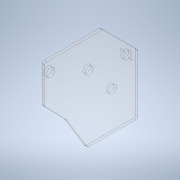
# Autodesk Inventor part: Intake-v2
Saved by Autodesk Inventor 2022 (Build 260153000, 153)
## iProperties
Created: 2022-01-09
Part Number: Intake-v2
Material: Generic
Document SubType Name: Modeling
Designer: merky
Density: 1 g/cm^3
Appearance: Polycarbonate - Clear
Mass: 272.104 g
Surface Area: 946.386 cm^2
Volume: 272.104 cm^3
Author: merky
Autodesk Inventor part; units mm, degrees
ref_plane "YZ Plane" through (0, 0, 0) normal (1, 0, 0) x (0, 1, 0)
ref_plane "XZ Plane" through (0, 0, 0) normal (0, 1, 0) x (-1, 0, 0)
ref_plane "XY Plane" through (0, 0, 0) normal (0, 0, 1) x (1, 0, 0)
sketch "Sketch1" plane through (0, 0, 0) normal (1, 0, 0) x (0, 1, 0)
  line L0 (348.73, -1.5913) -> (348.73, -164.0611)
  line L1 (346.8701, -168.5512) -> (220.7492, -294.6721)
  line L2 (216.2591, -296.532) -> (6.3382, -296.532)
  circle A0 centre (307.9632, 25.3963) radius 15.5575
  line L3 (348.73, -1.5913) -> (348.73, 40.2549)
  line L4 (-0.0118, -114.6125) -> (-0.0118, -290.182)
  arc A1 (5.4588, -108.3237) -> (-0.0118, -114.6125) centre (6.3382, -114.6125) ccw
  arc A2 (-0.0118, -290.182) -> (6.3382, -296.532) centre (6.3382, -290.182) ccw
  arc A3 (216.2591, -296.532) -> (220.7492, -294.6721) centre (216.2591, -290.182) ccw
  arc A4 (346.8701, -168.5512) -> (348.73, -164.0611) centre (342.38, -164.0611) ccw
  circle A5 centre (243.0455, -117.7246) radius 14.2875
  circle A6 centre (243.0455, -117.7246) radius 38.1 construction
  circle A7 centre (140.3051, -203.2037) radius 38.1 construction
  circle A8 centre (140.3051, -203.2037) radius 14.2875
  circle A9 centre (200.1626, -272.0217) radius 2.5781
  circle A10 centre (221.1605, -257.7302) radius 14.2875
  circle A11 centre (242.1584, -243.4386) radius 2.5781
  line L5 (207.9895, 44.8163) -> (126.5223, -34.0863)
  line L6 (125.4182, -34.9418) -> (5.4588, -108.3237)
  arc A12 (125.4182, -34.9418) -> (126.5223, -34.0863) centre (122.1046, -29.525) ccw
  line L7 (212.4073, 46.6049) -> (342.38, 46.6049)
  arc A13 (348.73, 40.2549) -> (342.38, 46.6049) centre (342.38, 40.2549) ccw
  arc A14 (212.4073, 46.6049) -> (207.9895, 44.8163) centre (212.4073, 40.2549) ccw
  point P0 (348.73, -166.6913)
  point P1 (182.4228, -257.7338)
  point P2 (269.24, 25.4)
  dimension "d49" = 28.575
  dimension "d50" = 76.2
  dimension "d51" = 76.2
  dimension "d52" = 28.575
  dimension "d53" = 28.575
  dimension "d54" = 5.1562
  dimension "d56" = 6.35
  constraints: 16 end point, 15 centre point, 14 point on circle, 13 tangent, 4 coincident, 2 perpendicular, 2 point on line, 1 equal radius, 1 vertical
  measures "d49" diameter of A5
  measures "d50" diameter of A6
  measures "d51" diameter of A7
  measures "d52" diameter of A8
  measures "d53" diameter of A10
  measures "d54" diameter of A11
  measures "d56" radius of A13
extrude "Extrusion1" add sketch "Sketch1" along normal blind 9.525
body "Solid1"
